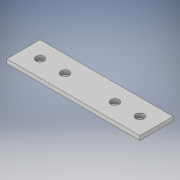
# Autodesk Inventor part: 1x4x0125 straight gusset
Saved by Autodesk Inventor 2017 (Build 210142000, 142)
## iProperties
Created: 2016-10-06
Part Number: 1x4x0125 straight gusset
Material: Generic
Document SubType Name: Modeling
Designer: 15102898
Density: 1 g/cm^3
Appearance: Default
Author: 15102898
Autodesk Inventor part; units mm, degrees
ref_plane "YZ Plane" through (0, 0, 0) normal (1, 0, 0) x (0, 1, 0)
ref_plane "XZ Plane" through (0, 0, 0) normal (0, 1, 0) x (-1, 0, 0)
ref_plane "XY Plane" through (0, 0, 0) normal (0, 0, 1) x (1, 0, 0)
sketch "Sketch1" plane through (0, 0, 0) normal (0, 1, 0) x (-1, 0, 0)
  line L0 (0, 0) -> (101.6, 0)
  line L1 (101.6, 0) -> (101.6, 25.4)
  line L2 (101.6, 25.4) -> (0, 25.4)
  line L3 (0, 25.4) -> (0, 0)
  circle A0 centre (88.9, 12.7) radius 3.175
  circle A1 centre (69.85, 12.7) radius 3.175
  circle A2 centre (31.75, 12.7) radius 3.175
  circle A3 centre (12.7, 12.7) radius 3.175
  dimension "d0" = 101.6
  dimension "d1" = 25.4
  dimension "d2" = 12.7
  dimension "d3" = 12.7
  dimension "d4" = 19.05
  dimension "d5" = 12.7
  dimension "d6" = 12.7
  dimension "d7" = 12.7
  dimension "d8" = 19.05
  dimension "d9" = 12.7
  dimension "d10" = 6.35
  dimension "d11" = 6.35
  dimension "d12" = 6.35
  dimension "d13" = 6.35
  constraints: 8 end point, 4 centre point, 4 coincident, 2 parallel, 1 horizontal, 1 perpendicular
  measures "d0" distance of L2.end L1.end
  measures "d1" distance of L2.end L0.start
  measures "d2" distance from line of L1 point (88.9, 12.7)
  measures "d3" distance from line of L0 point (88.9, 12.7)
  measures "d4" distance of point (88.9, 12.7) point (69.85, 12.7)
  measures "d5" distance from line of L0 point (69.85, 12.7)
  measures "d6" distance from line of L3 point (12.7, 12.7)
  measures "d7" distance from line of L0 point (12.7, 12.7)
  measures "d8" distance of point (12.7, 12.7) point (31.75, 12.7)
  measures "d9" distance from line of L0 point (31.75, 12.7)
  measures "d10" diameter of A0
  measures "d11" diameter of A1
  measures "d12" diameter of A2
  measures "d13" diameter of A3
extrude "Extrusion1" add sketch "Sketch1" along normal blind 3.175
body "Solid1"
